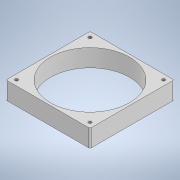
# Autodesk Inventor part: Lüfter80x80
Saved by Autodesk Inventor 2021.3 (Build 253353000, 353)
## iProperties
Created: 2021-10-11
Part Number: Lüfter80x80
Material: Generisch
Document SubType Name: Modeling
Designer: bhelg
Density: 1 g/cm^3
Appearance: Vorgabe
Author: bhelg
Autodesk Inventor part; units mm, degrees
ref_plane "YZ Plane" through (0, 0, 0) normal (1, 0, 0) x (0, 1, 0)
ref_plane "XZ Plane" through (0, 0, 0) normal (0, 1, 0) x (-1, 0, 0)
ref_plane "XY Plane" through (0, 0, 0) normal (0, 0, 1) x (1, 0, 0)
sketch "Skizze1" plane through (0, 0, 0) normal (0, 1, 0) x (-1, 0, 0)
  line L0 (-60, -60) -> (60, -60)
  line L1 (60, -60) -> (60, 60)
  line L2 (60, 60) -> (-60, 60)
  line L3 (-60, 60) -> (-60, -60)
  line L4 (-60, -60) -> (60, 60) construction
  line L5 (60, -60) -> (-60, 60) construction
  point P0 (0, 0)
  dimension "d0" = 120
  dimension "d1" = 120
  constraints: 12 end point, 2 midpoint, 2 parallel, 1 horizontal, 1 perpendicular
  measures "d0" distance of L0.end L1.end
  measures "d1" distance of L1.end L2.end
extrude "Extrusion1" add sketch "Skizze1" along normal blind 25
sketch "Skizze2" plane through (0, 25, 0) normal (0, 1, 0) x (1, 0, 0)
  line L0 (52.5, 52.5) -> (-52.5, 52.5)
  line L1 (-52.5, 52.5) -> (-52.5, -52.5)
  line L2 (-52.5, -52.5) -> (52.5, -52.5)
  line L3 (52.5, -52.5) -> (52.5, 52.5)
  line L4 (52.5, 52.5) -> (-52.5, -52.5) construction
  line L5 (-52.5, 52.5) -> (52.5, -52.5) construction
  point P0 (0, 0)
  dimension "d4" = 105
  dimension "d5" = 105
  constraints: 12 end point, 2 midpoint, 2 parallel, 1 horizontal, 1 perpendicular
  measures "d4" distance of L0.end L1.end
  measures "d5" distance of L1.end L2.end
hole "Bohrung1" at (52.5, 25, 52.5) at (52.5, 25, -52.5) at (-52.5, 25, 52.5) at (-52.5, 25, -52.5) direction (0, -1, 0) diameter 4.3 end through all
sketch "Skizze3" plane through (0, 25, 0) normal (0, 1, 0) x (1, 0, 0)
  circle A0 centre (0, 0) radius 56.5
  dimension "d13" = 113
  constraints: 1 centre point, 1 coincident
  measures "d13" diameter of A0
extrude "Extrusion2" cut sketch "Skizze3" against normal through all
fillet "Rundung1" radius 2 4 edges at (-60, 12.5, 60) (60, 12.5, 60) (-60, 12.5, -60) (60, 12.5, -60)
